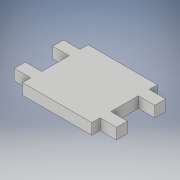
# Autodesk Inventor part: wall-back-scaled
Saved by Autodesk Inventor 2017 (Build 210142000, 142)
## iProperties
Created: 2017-02-28
Part Number: wall-back-scaled
Material: Generic
Document SubType Name: Modeling
Designer: John
Density: 1 g/cm^3
Appearance: Default
Author: John
Autodesk Inventor part; units mm, degrees
ref_plane "YZ Plane" through (0, 0, 0) normal (1, 0, 0) x (0, 1, 0)
ref_plane "XZ Plane" through (0, 0, 0) normal (0, 1, 0) x (-1, 0, 0)
ref_plane "XY Plane" through (0, 0, 0) normal (0, 0, 1) x (1, 0, 0)
sketch "Sketch1" plane through (0, 0, 0) normal (0, 1, 0) x (-1, 0, 0)
  line L0 (19, -18) -> (-19, -18)
  line L1 (-19, -18) -> (-19, 18)
  line L2 (-19, 18) -> (19, 18)
  line L3 (19, 18) -> (19, -18)
  line L4 (19, -18) -> (-19, 18) construction
  line L5 (-19, -18) -> (19, 18) construction
  line L6 (-19, 13.5) -> (-28, 13.5)
  line L7 (-28, 13.5) -> (-28, 7.5)
  line L8 (-28, 7.5) -> (-19, 7.5)
  line L9 (-19, 7.5) -> (-19, 13.5)
  line L10 (-19, -7.5) -> (-28, -7.5)
  line L11 (-28, -7.5) -> (-28, -13.5)
  line L12 (-28, -13.5) -> (-19, -13.5)
  line L13 (-19, -13.5) -> (-19, -7.5)
  line L14 (0, 18) -> (0, -18) construction
  line L15 (19, 13.5) -> (28, 13.5)
  line L16 (28, 13.5) -> (28, 7.5)
  line L17 (28, 7.5) -> (19, 7.5)
  line L18 (19, 7.5) -> (19, 13.5)
  line L19 (19, -7.5) -> (28, -7.5)
  line L20 (28, -7.5) -> (28, -13.5)
  line L21 (28, -13.5) -> (19, -13.5)
  line L22 (19, -13.5) -> (19, -7.5)
  point P0 (0, 0)
  dimension "d0" = 38
  dimension "d1" = 36
  dimension "d2" = 9
  dimension "d3" = 6
  dimension "d4" = 9
  dimension "d5" = 6
  dimension "d6" = 4.5
  dimension "d7" = 15
  constraints: 46 end point, 8 symmetric about line, 6 parallel, 4 midpoint, 3 horizontal, 3 perpendicular, 2 point on line
  measures "d0" distance of L1.end L2.end
  measures "d1" distance of L0.end L1.end
  measures "d2" distance of L8.end L7.end
  measures "d3" distance of L7.end L6.end
  measures "d4" distance of L12.end L11.end
  measures "d5" distance of L11.end L10.end
  measures "d6" distance between parallel lines of L0 L12
  measures "d7" distance between parallel lines of L8 L10
extrude "Extrusion1" add sketch "Sketch1" along normal blind 6
body "Solid1"
